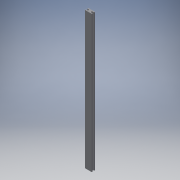
# Autodesk Inventor part: Riel
Saved by Autodesk Inventor 2018 (Build 220112000, 112)
## iProperties
Created: 2021-07-09
Part Number: Riel
Material: Genérico
Document SubType Name: Modeling
Designer: GABRIEL
Density: 1 g/cm^3
Appearance: Valor por defecto
Author: GABRIEL
Autodesk Inventor part; units mm, degrees
ref_plane "YZ Plane" through (0, 0, 0) normal (1, 0, 0) x (0, 1, 0)
ref_plane "XZ Plane" through (0, 0, 0) normal (0, 1, 0) x (-1, 0, 0)
ref_plane "XY Plane" through (0, 0, 0) normal (0, 0, 1) x (1, 0, 0)
sketch "Boceto1" plane through (0, 0, 0) normal (0, 0, 1) x (1, 0, 0)
  line L0 (0, 0) -> (10, 0)
  line L1 (10, 0) -> (10, -1.5)
  line L2 (10, -1.5) -> (7, -1.5)
  line L3 (7, -1.5) -> (7, -3.5)
  line L4 (7, -3.5) -> (10, -3.5)
  line L5 (10, -3.5) -> (10, -5)
  line L6 (10, -5) -> (0, -5)
  line L7 (0, -5) -> (0, -3.5)
  line L8 (0, -3.5) -> (3, -3.5)
  line L9 (0, -1.5) -> (0, 0)
  line L10 (0, -1.5) -> (3, -1.5)
  line L11 (3, -1.5) -> (3, -3.5)
  dimension "d0" = 10
  dimension "d1" = 1.5
  dimension "d2" = 3
  dimension "d3" = 2
  dimension "d4" = 1.5
  dimension "d5" = 1.5
  dimension "d6" = 3
  dimension "d7" = 3
  constraints: 24 end point, 6 perpendicular, 6 point on line, 2 horizontal
  measures "d0" distance of L0.start L0.end
  measures "d1" distance of L0.end L1.end
  measures "d2" distance of L1.end L2.end
  measures "d3" distance of L2.end L3.end
  measures "d4" distance of L4.end L5.end
  measures "d5" distance of L6.end L7.end
  measures "d6" distance of L7.end L8.end
  measures "d7" distance of L9.start L10.end
extrude "Extrusión1" add sketch "Boceto1" along normal blind 120
